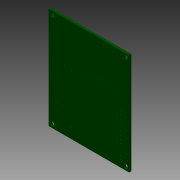
# Autodesk Inventor part: MSP-EXP430F5529LP
Saved by Autodesk Inventor 2015 SP1 (Build 190203100, 203)
## iProperties
Category: Control System
Company: Autodesk Inc.
Created: 2014-12-18
Part Number: MSP-EXP430F5529LP
Material: Generic
Document SubType Name: Modeling
Designer: Autodesk Inc.
Density: 1 g/cm^3
Appearance: Board Outline
Catalog Web Link: http://www.ti.com/tool/msp-exp430f5529lp
Vendor: Texas Instruments
Author: Autodesk Inc.
Autodesk Inventor part; units mm, degrees
ref_plane "YZ Plane" through (0, 0, 0) normal (1, 0, 0) x (0, 1, 0)
ref_plane "XZ Plane" through (0, 0, 0) normal (0, 1, 0) x (-1, 0, 0)
ref_plane "XY Plane" through (0, 0, 0) normal (0, 0, 1) x (1, 0, 0)
sketch "Sketch1" plane through (0, 0, 0) normal (0, 0, 1) x (1, 0, 0)
  line L0 (-3.81, 73.66) -> (-3.81, 0)
  line L1 (-3.81, 0) -> (54.61, 0)
  line L2 (54.61, 0) -> (54.61, 73.66)
  line L3 (54.61, 73.66) -> (-3.81, 73.66)
  circle A0 centre (2.54, 35.56) radius 0.455
  circle A1 centre (5.08, 35.56) radius 0.455
  circle A2 centre (2.54, 33.02) radius 0.455
  circle A3 centre (5.08, 33.02) radius 0.455
  circle A4 centre (2.54, 30.48) radius 0.455
  circle A5 centre (5.08, 30.48) radius 0.455
  circle A6 centre (2.54, 27.94) radius 0.455
  circle A7 centre (5.08, 27.94) radius 0.455
  circle A8 centre (2.54, 25.4) radius 0.455
  circle A9 centre (5.08, 25.4) radius 0.455
  circle A10 centre (2.54, 22.86) radius 0.455
  circle A11 centre (5.08, 22.86) radius 0.455
  circle A12 centre (2.54, 20.32) radius 0.455
  circle A13 centre (5.08, 20.32) radius 0.455
  circle A14 centre (2.54, 17.78) radius 0.455
  circle A15 centre (5.08, 17.78) radius 0.455
  circle A16 centre (2.54, 15.24) radius 0.455
  circle A17 centre (5.08, 15.24) radius 0.455
  circle A18 centre (2.54, 12.7) radius 0.455
  circle A19 centre (5.08, 12.7) radius 0.455
  circle A20 centre (2.54, 7.62) radius 0.455
  circle A21 centre (2.54, 5.08) radius 0.455
  circle A22 centre (2.54, 2.54) radius 0.455
  circle A23 centre (45.72, 35.56) radius 0.455
  circle A24 centre (48.26, 35.56) radius 0.455
  circle A25 centre (45.72, 33.02) radius 0.455
  circle A26 centre (48.26, 33.02) radius 0.455
  circle A27 centre (45.72, 30.48) radius 0.455
  circle A28 centre (48.26, 30.48) radius 0.455
  circle A29 centre (45.72, 27.94) radius 0.455
  circle A30 centre (48.26, 27.94) radius 0.455
  circle A31 centre (45.72, 25.4) radius 0.455
  circle A32 centre (48.26, 25.4) radius 0.455
  circle A33 centre (45.72, 22.86) radius 0.455
  circle A34 centre (48.26, 22.86) radius 0.455
  circle A35 centre (45.72, 20.32) radius 0.455
  circle A36 centre (48.26, 20.32) radius 0.455
  circle A37 centre (45.72, 17.78) radius 0.455
  circle A38 centre (48.26, 17.78) radius 0.455
  circle A39 centre (45.72, 15.24) radius 0.455
  circle A40 centre (48.26, 15.24) radius 0.455
  circle A41 centre (45.72, 12.7) radius 0.455
  circle A42 centre (48.26, 12.7) radius 0.455
  circle A43 centre (48.26, 7.62) radius 0.455
  circle A44 centre (48.26, 5.08) radius 0.455
  circle A45 centre (48.26, 2.54) radius 0.455
  circle A46 centre (27.94, 48.26) radius 0.455
  circle A47 centre (27.94, 45.72) radius 0.455
  circle A48 centre (30.48, 48.26) radius 0.455
  circle A49 centre (30.48, 45.72) radius 0.455
  circle A50 centre (25.4, 45.72) radius 0.455
  circle A51 centre (25.4, 48.26) radius 0.455
  circle A52 centre (45.72, 48.26) radius 0.455
  circle A53 centre (45.72, 45.72) radius 0.455
  circle A54 centre (43.18, 48.26) radius 0.455
  circle A55 centre (43.18, 45.72) radius 0.455
  circle A56 centre (48.26, 48.26) radius 0.455
  circle A57 centre (48.26, 45.72) radius 0.455
  circle A58 centre (40.64, 48.26) radius 0.455
  circle A59 centre (40.64, 45.72) radius 0.455
  circle A60 centre (38.1, 48.26) radius 0.455
  circle A61 centre (38.1, 45.72) radius 0.455
  circle A62 centre (35.56, 48.26) radius 0.455
  circle A63 centre (35.56, 45.72) radius 0.455
  circle A64 centre (33.02, 48.29) radius 0.455
  circle A65 centre (33.02, 45.75) radius 0.455
  circle A66 centre (25.4, 5.08) radius 0.455
  circle A67 centre (25.4, 2.54) radius 0.455
  circle A68 centre (12.7, 7.62) radius 0.51
  circle A69 centre (12.7, 2.62) radius 0.51
  circle A70 centre (38.1, 7.62) radius 0.51
  circle A71 centre (38.1, 2.62) radius 0.51
  circle A72 centre (2.54, 43.18) radius 0.51
  circle A73 centre (7.54, 43.18) radius 0.51
  circle A74 centre (12.7, 43.18) radius 0.51
  circle A75 centre (17.7, 43.18) radius 0.51
  circle A76 centre (48.26, 71.12) radius 0.455
  circle A77 centre (45.72, 71.12) radius 0.455
  circle A78 centre (43.18, 71.12) radius 0.455
  circle A79 centre (40.64, 71.12) radius 0.455
  circle A80 centre (38.1, 71.12) radius 0.455
  circle A81 centre (35.56, 71.12) radius 0.455
  circle A82 centre (33.02, 71.12) radius 0.455
  circle A83 centre (-1.27, 71.12) radius 1.5875
  circle A84 centre (52.07, 71.12) radius 1.5875
  circle A85 centre (52.07, 2.54) radius 1.5875
  circle A86 centre (-1.27, 2.54) radius 1.5875
  circle A87 centre (17.9832, 60.833) radius 0.1524
  circle A88 centre (20.6248, 63.246) radius 0.1524
  circle A89 centre (15.367, 60.7314) radius 0.1524
  circle A90 centre (24.0538, 66.3448) radius 0.1524
  circle A91 centre (17.526, 59.8932) radius 0.1524
  circle A92 centre (20.0406, 61.2394) radius 0.1524
  circle A93 centre (14.2748, 61.087) radius 0.1524
  circle A94 centre (21.59, 62.865) radius 0.1524
  circle A95 centre (25.019, 65.786) radius 0.1524
  circle A96 centre (35.941, 25.4762) radius 0.1524
  circle A97 centre (22.86, 39.9542) radius 0.1524
  circle A98 centre (25.7302, 42.2656) radius 0.1524
  circle A99 centre (16.5354, 15.0114) radius 0.1524
  circle A100 centre (38.4048, 17.018) radius 0.1524
  circle A101 centre (16.764, 22.5044) radius 0.1524
  circle A102 centre (5.3848, 10.4648) radius 0.1524
  circle A103 centre (10.414, 10.5156) radius 0.1524
  circle A104 centre (38.2778, 10.8712) radius 0.1524
  circle A105 centre (23.6982, 39.1668) radius 0.1524
  circle A106 centre (25.8826, 41.0718) radius 0.1524
  circle A107 centre (7.1628, 39.878) radius 0.1524
  circle A108 centre (7.1628, 37.6682) radius 0.1524
  circle A109 centre (26.4414, 63.4238) radius 0.1524
  circle A110 centre (28.9052, 62.103) radius 0.1524
  circle A111 centre (32.7152, 54.8386) radius 0.1524
  circle A112 centre (30.8356, 57.404) radius 0.1524
  circle A113 centre (25.7302, 62.5348) radius 0.1524
  circle A114 centre (28.5242, 61.214) radius 0.1524
  circle A115 centre (31.7754, 54.0258) radius 0.1524
  circle A116 centre (29.972, 56.4896) radius 0.1524
  circle A117 centre (17.5768, 50.4444) radius 0.1524
  circle A118 centre (19.6088, 52.451) radius 0.1524
  circle A119 centre (38.4556, 63.754) radius 0.1524
  circle A120 centre (40.4114, 59.9186) radius 0.1524
  circle A121 centre (41.6814, 58.6232) radius 0.1524
  circle A122 centre (38.7096, 61.6204) radius 0.1524
  circle A123 centre (38.7858, 52.4764) radius 0.1524
  circle A124 centre (36.068, 51.6128) radius 0.1524
  circle A125 centre (32.258, 52.4764) radius 0.1524
  circle A126 centre (27.432, 52.451) radius 0.1524
  circle A127 centre (29.591, 52.4764) radius 0.1524
  circle A128 centre (31.0134, 51.2572) radius 0.1524
  circle A129 centre (16.7386, 51.308) radius 0.1524
  circle A130 centre (18.9992, 53.5178) radius 0.1524
  circle A131 centre (43.7134, 52.1208) radius 0.1524
  circle A132 centre (28.3718, 70.5612) radius 0.1524
  circle A133 centre (42.5704, 50.1142) radius 0.1524
  circle A134 centre (36.2966, 50.5714) radius 0.1524
  circle A135 centre (28.4734, 68.6308) radius 0.1524
  circle A136 centre (30.2768, 66.7512) radius 0.1524
  circle A137 centre (30.5562, 62.103) radius 0.1524
  circle A138 centre (7.0866, 55.4736) radius 0.1524
  circle A139 centre (11.557, 64.5922) radius 0.1524
  circle A140 centre (20.066, 67.5132) radius 0.1524
  circle A141 centre (13.97, 67.4116) radius 0.1524
  circle A142 centre (12.573, 67.4116) radius 0.1524
  circle A143 centre (13.1826, 62.484) radius 0.1524
  circle A144 centre (13.1826, 60.5536) radius 0.1524
  circle A145 centre (7.2898, 66.0146) radius 0.1524
  circle A146 centre (6.7818, 64.516) radius 0.1524
  circle A147 centre (7.3914, 68.2244) radius 0.1524
  circle A148 centre (3.6576, 66.9798) radius 0.1524
  circle A149 centre (6.0452, 58.42) radius 0.1524
  circle A150 centre (4.064, 54.2544) radius 0.1524
  circle A151 centre (28.3718, 59.9694) radius 0.1524
  circle A152 centre (11.557, 63.4746) radius 0.1524
  circle A153 centre (23.1902, 69.6468) radius 0.1524
  circle A154 centre (27.3812, 69.6468) radius 0.1524
  circle A155 centre (28.3464, 71.7042) radius 0.1524
  circle A156 centre (42.6212, 5.715) radius 0.1524
  circle A157 centre (7.6962, 5.1308) radius 0.1524
  circle A158 centre (22.1234, 1.9304) radius 0.1524
  circle A159 centre (32.1564, 1.905) radius 0.1524
  circle A160 centre (16.9418, 19.2786) radius 0.1524
  circle A161 centre (11.0744, 24.5618) radius 0.1524
  circle A162 centre (32.893, 58.8772) radius 0.1524
  circle A163 centre (34.4678, 62.6872) radius 0.1524
  circle A164 centre (31.9786, 61.9506) radius 0.1524
  circle A165 centre (42.799, 51.2318) radius 0.1524
  circle A166 centre (45.8216, 61.6712) radius 0.1524
  circle A167 centre (44.958, 62.5094) radius 0.1524
  circle A168 centre (11.5062, 67.7164) radius 0.1524
  circle A169 centre (14.7066, 57.7088) radius 0.1524
  circle A170 centre (18.288, 57.7342) radius 0.1524
  circle A171 centre (18.288, 56.3118) radius 0.1524
  circle A172 centre (14.7066, 56.3118) radius 0.1524
  circle A173 centre (30.8102, 32.2326) radius 0.1524
  circle A174 centre (28.1432, 37.7444) radius 0.1524
  circle A175 centre (26.797, 37.7444) radius 0.1524
  circle A176 centre (26.6192, 30.6324) radius 0.1524
  circle A177 centre (23.5712, 38.2016) radius 0.1524
  circle A178 centre (34.3154, 32.639) radius 0.1524
  circle A179 centre (35.8902, 24.1554) radius 0.1524
  circle A180 centre (19.685, 44.6532) radius 0.1524
  circle A181 centre (23.4188, 44.6786) radius 0.1524
  circle A182 centre (20.3962, 42.5196) radius 0.1524
  circle A183 centre (10.4902, 45.7454) radius 0.1524
  circle A184 centre (21.0058, 13.3096) radius 0.1524
  circle A185 centre (18.5928, 15.3924) radius 0.1524
  circle A186 centre (14.4272, 18.6944) radius 0.1524
  circle A187 centre (10.9728, 18.6944) radius 0.1524
  circle A188 centre (45.8978, 63.3222) radius 0.1524
  circle A189 centre (48.9966, 58.9534) radius 0.1524
  circle A190 centre (45.1612, 57.3024) radius 0.1524
  circle A191 centre (45.6692, 55.6768) radius 0.1524
  circle A192 centre (34.544, 66.2432) radius 0.1524
  circle A193 centre (30.3784, 54.1274) radius 0.1524
  circle A194 centre (38.6842, 60.0456) radius 0.1524
  circle A195 centre (35.7378, 57.0992) radius 0.1524
  circle A196 centre (37.5666, 55.2704) radius 0.1524
  circle A197 centre (41.5798, 57.0484) radius 0.1524
  circle A198 centre (40.6146, 57.9628) radius 0.1524
  circle A199 centre (39.6748, 58.9026) radius 0.1524
  circle A200 centre (37.7444, 59.0804) radius 0.1524
  circle A201 centre (36.7792, 58.0898) radius 0.1524
  circle A202 centre (38.608, 58.0898) radius 0.1524
  circle A203 centre (37.6428, 57.0738) radius 0.1524
  circle A204 centre (36.6522, 56.2356) radius 0.1524
  circle A205 centre (38.6334, 54.1274) radius 0.1524
  circle A206 centre (39.5732, 55.0926) radius 0.1524
  circle A207 centre (40.6146, 56.134) radius 0.1524
  circle A208 centre (39.6748, 57.0738) radius 0.1524
  circle A209 centre (38.6334, 56.0832) radius 0.1524
  circle A210 centre (45.6184, 66.8782) radius 0.1524
  circle A211 centre (43.3578, 63.7032) radius 0.1524
  circle A212 centre (42.037, 63.6016) radius 0.1524
  circle A213 centre (31.8008, 65.5828) radius 0.1524
  circle A214 centre (24.2316, 68.3514) radius 0.1524
  circle A215 centre (24.2316, 67.2592) radius 0.1524
  circle A216 centre (24.2824, 63.8556) radius 0.1524
  circle A217 centre (24.2824, 64.9732) radius 0.1524
  circle A218 centre (22.1742, 61.341) radius 0.1524
  circle A219 centre (23.5458, 61.341) radius 0.1524
  circle A220 centre (23.4696, 57.7596) radius 0.1524
  circle A221 centre (22.1234, 57.7596) radius 0.1524
  circle A222 centre (12.5476, 69.9516) radius 0.1524
  circle A223 centre (17.7292, 68.0466) radius 0.1524
  circle A224 centre (16.4338, 68.6054) radius 0.1524
  circle A225 centre (2.3114, 55.245) radius 0.1524
  circle A226 centre (-1.4478, 38.1254) radius 0.1524
  circle A227 centre (-2.3622, 43.1546) radius 0.1524
  circle A228 centre (-0.4826, 48.5902) radius 0.1524
  circle A229 centre (5.0292, 45.7454) radius 0.1524
  circle A230 centre (15.1892, 45.6184) radius 0.1524
  circle A231 centre (15.8242, 40.5384) radius 0.1524
  circle A232 centre (43.1292, 10.9474) radius 0.1524
  circle A233 centre (10.6426, 35.4584) radius 0.1524
  circle A234 centre (14.4272, 36.0934) radius 0.1524
  circle A235 centre (17.526, 36.2204) radius 0.1524
  circle A236 centre (24.5872, 33.6804) radius 0.1524
  circle A237 centre (20.2184, 29.6418) radius 0.1524
  circle A238 centre (23.9522, 29.6164) radius 0.1524
  circle A239 centre (22.1488, 26.5938) radius 0.1524
  circle A240 centre (37.2872, 23.7744) radius 0.1524
  circle A241 centre (29.4132, 26.9494) radius 0.1524
  circle A242 centre (31.0642, 34.6964) radius 0.1524
  circle A243 centre (28.0162, 41.1734) radius 0.1524
  circle A244 centre (31.6992, 43.9674) radius 0.1524
  circle A245 centre (41.9354, 34.1122) radius 0.1524
  circle A246 centre (48.0568, 38.0746) radius 0.1524
  circle A247 centre (33.4772, 31.7754) radius 0.1524
  circle A248 centre (34.3408, 41.529) radius 0.1524
  circle A249 centre (34.3408, 37.2872) radius 0.1524
  circle A250 centre (41.0972, 37.3634) radius 0.1524
  circle A251 centre (39.7002, 42.4434) radius 0.1524
  circle A252 centre (47.0662, 43.5864) radius 0.1524
  circle A253 centre (44.5262, 39.0144) radius 0.1524
  circle A254 centre (43.2054, 31.8008) radius 0.1524
  circle A255 centre (50.8762, 37.1094) radius 0.1524
  circle A256 centre (50.546, 49.6316) radius 0.1524
  circle A257 centre (46.8884, 53.6702) radius 0.1524
  circle A258 centre (50.6222, 53.6194) radius 0.1524
  circle A259 centre (49.9872, 56.6674) radius 0.1524
  circle A260 centre (50.4952, 60.7314) radius 0.1524
  circle A261 centre (50.6222, 65.4304) radius 0.1524
  circle A262 centre (49.8602, 67.7164) radius 0.1524
  circle A263 centre (50.4952, 63.0174) radius 0.1524
  circle A264 centre (46.5582, 66.1924) radius 0.1524
  circle A265 centre (39.3192, 66.0654) radius 0.1524
  circle A266 centre (39.1922, 67.7164) radius 0.1524
  circle A267 centre (37.7952, 67.8434) radius 0.1524
  circle A268 centre (32.8422, 67.4624) radius 0.1524
  circle A269 centre (31.5722, 66.8274) radius 0.1524
  circle A270 centre (35.7632, 62.2554) radius 0.1524
  circle A271 centre (38.5318, 66.8274) radius 0.1524
  circle A272 centre (36.7792, 70.1294) radius 0.1524
  circle A273 centre (41.8592, 70.1294) radius 0.1524
  circle A274 centre (21.6662, 72.1614) radius 0.1524
  circle A275 centre (21.2852, 70.0024) radius 0.1524
  circle A276 centre (24.4602, 62.5094) radius 0.1524
  circle A277 centre (26.6192, 56.6674) radius 0.1524
  circle A278 centre (27.5082, 67.7164) radius 0.1524
  circle A279 centre (26.8732, 58.4454) radius 0.1524
  circle A280 centre (22.8092, 54.6354) radius 0.1524
  circle A281 centre (23.4442, 55.6514) radius 0.1524
  circle A282 centre (19.6342, 57.8104) radius 0.1524
  circle A283 centre (19.8882, 54.7624) radius 0.1524
  circle A284 centre (23.4696, 51.6128) radius 0.1524
  circle A285 centre (20.9042, 51.4604) radius 0.1524
  circle A286 centre (46.9392, 50.3936) radius 0.1524
  circle A287 centre (17.3482, 48.9204) radius 0.1524
  circle A288 centre (18.8722, 48.0314) radius 0.1524
  circle A289 centre (26.7462, 54.6354) radius 0.1524
  circle A290 centre (19.7612, 45.9994) radius 0.1524
  circle A291 centre (18.5928, 46.355) radius 0.1524
  circle A292 centre (15.5702, 49.3014) radius 0.1524
  circle A293 centre (14.0462, 49.5554) radius 0.1524
  circle A294 centre (14.3002, 52.2224) radius 0.1524
  circle A295 centre (16.2052, 52.4764) radius 0.1524
  circle A296 centre (13.6652, 53.4924) radius 0.1524
  circle A297 centre (13.0302, 56.5404) radius 0.1524
  circle A298 centre (10.6172, 59.5884) radius 0.1524
  circle A299 centre (9.7282, 58.5724) radius 0.1524
  circle A300 centre (8.4582, 58.1914) radius 0.1524
  circle A301 centre (9.2202, 59.8424) radius 0.1524
  circle A302 centre (9.2202, 61.4934) radius 0.1524
  circle A303 centre (8.7122, 62.8904) radius 0.1524
  circle A304 centre (6.9342, 62.5094) radius 0.1524
  circle A305 centre (5.5372, 62.5094) radius 0.1524
  circle A306 centre (4.3942, 62.2554) radius 0.1524
  circle A307 centre (3.5052, 61.3664) radius 0.1524
  circle A308 centre (3.5052, 60.0964) radius 0.1524
  circle A309 centre (19.6342, 72.6694) radius 0.1524
  circle A310 centre (13.0302, 68.8594) radius 0.1524
  circle A311 centre (13.7922, 72.7964) radius 0.1524
  circle A312 centre (1.3462, 61.4934) radius 0.1524
  circle A313 centre (1.3462, 59.9694) radius 0.1524
  circle A314 centre (1.905, 69.9516) radius 0.1524
  circle A315 centre (-2.2606, 53.975) radius 0.1524
  circle A316 centre (-2.4638, 56.9214) radius 0.1524
  circle A317 centre (0.635, 67.8434) radius 0.1524
  circle A318 centre (-0.2794, 66.4972) radius 0.1524
  circle A319 centre (-2.0066, 50.1396) radius 0.1524
  circle A320 centre (-1.2192, 60.6806) radius 0.1524
  circle A321 centre (-0.1778, 64.9986) radius 0.1524
  circle A322 centre (-0.5588, 55.9054) radius 0.1524
  circle A323 centre (-0.4826, 53.8988) radius 0.1524
  circle A324 centre (-0.5334, 52.2224) radius 0.1524
  circle A325 centre (-0.254, 50.6476) radius 0.1524
  circle A326 centre (0.8382, 49.4284) radius 0.1524
  circle A327 centre (6.5532, 49.4284) radius 0.1524
  circle A328 centre (11.2522, 49.3014) radius 0.1524
  circle A329 centre (-1.0668, 34.0614) radius 0.1524
  circle A330 centre (-0.3048, 46.0502) radius 0.1524
  circle A331 centre (-1.0668, 31.6484) radius 0.1524
  circle A332 centre (-1.0668, 28.9814) radius 0.1524
  circle A333 centre (-1.1938, 26.5684) radius 0.1524
  circle A334 centre (-1.0668, 23.9014) radius 0.1524
  circle A335 centre (-1.1938, 21.717) radius 0.1524
  circle A336 centre (-1.1176, 19.1008) radius 0.1524
  circle A337 centre (-1.016, 16.4084) radius 0.1524
  circle A338 centre (-1.3208, 13.7668) radius 0.1524
  circle A339 centre (-0.3048, 10.5664) radius 0.1524
  circle A340 centre (0.7112, 9.2964) radius 0.1524
  circle A341 centre (6.223, 9.017) radius 0.1524
  circle A342 centre (18.6944, 9.9822) radius 0.1524
  circle A343 centre (46.5582, 6.3754) radius 0.1524
  circle A344 centre (49.7332, 10.3124) radius 0.1524
  circle A345 centre (51.8922, 11.2014) radius 0.1524
  circle A346 centre (51.5112, 13.8684) radius 0.1524
  circle A347 centre (51.1302, 16.4084) radius 0.1524
  circle A348 centre (51.1302, 18.6944) radius 0.1524
  circle A349 centre (51.0032, 21.4884) radius 0.1524
  circle A350 centre (51.0032, 24.0284) radius 0.1524
  circle A351 centre (51.1302, 26.8224) radius 0.1524
  circle A352 centre (51.0032, 28.9814) radius 0.1524
  circle A353 centre (51.0032, 31.6484) radius 0.1524
  circle A354 centre (51.0032, 34.0614) radius 0.1524
  circle A355 centre (43.0022, 16.5354) radius 0.1524
  circle A356 centre (33.4772, 27.0764) radius 0.1524
  circle A357 centre (37.0332, 26.3144) radius 0.1524
  circle A358 centre (34.4932, 18.5674) radius 0.1524
  circle A359 centre (27.7622, 27.7114) radius 0.1524
  circle A360 centre (27.2796, 20.5994) radius 0.1524
  circle A361 centre (48.8442, 40.3352) radius 0.1524
  circle A362 centre (20.2438, 11.9126) radius 0.1524
  circle A363 centre (28.8544, 20.0914) radius 0.1524
  circle A364 centre (21.4884, 21.5392) radius 0.1524
  circle A365 centre (22.1488, 23.3426) radius 0.1524
  circle A366 centre (31.9278, 18.542) radius 0.1524
  circle A367 centre (42.8752, 23.9014) radius 0.1524
  circle A368 centre (17.2212, 17.6784) radius 0.1524
  circle A369 centre (19.5072, 14.7574) radius 0.1524
  circle A370 centre (14.1986, 13.8176) radius 0.1524
  circle A371 centre (17.2212, 4.4704) radius 0.1524
  circle A372 centre (9.779, 1.2954) radius 0.1524
  circle A373 centre (27.6352, 2.5654) radius 0.1524
  circle A374 centre (34.1122, 3.5814) radius 0.1524
  circle A375 centre (27.813, 6.0198) radius 0.1524
  circle A376 centre (40.0812, 5.1054) radius 0.1524
  circle A377 centre (9.0932, 36.7284) radius 0.1524
  circle A378 centre (53.2892, 6.5024) radius 0.1524
  circle A379 centre (-2.7178, 6.8834) radius 0.1524
  circle A380 centre (12.8016, 15.2146) radius 0.1524
  circle A381 centre (11.0998, 15.5448) radius 0.1524
  circle A382 centre (14.605, 15.7226) radius 0.1524
  circle A383 centre (14.6812, 17.2974) radius 0.1524
  circle A384 centre (12.7254, 20.32) radius 0.1524
  circle A385 centre (11.176, 17.3228) radius 0.1524
  circle A386 centre (15.1892, 22.6314) radius 0.1524
  circle A387 centre (23.4442, 33.6804) radius 0.1524
  circle A388 centre (1.4224, 31.7246) radius 0.1524
  circle A389 centre (30.3022, 39.3954) radius 0.1524
  circle A390 centre (33.2232, 34.0614) radius 0.1524
  circle A391 centre (15.367, 10.0076) radius 0.1524
  circle A392 centre (15.7734, 64.7192) radius 0.1524
  circle A393 centre (18.2626, 64.7192) radius 0.1524
  circle A394 centre (17.018, 64.7192) radius 0.1524
  circle A395 centre (15.7734, 65.9638) radius 0.1524
  circle A396 centre (18.2626, 65.9638) radius 0.1524
  circle A397 centre (17.018, 65.9638) radius 0.1524
  circle A398 centre (15.7734, 63.4492) radius 0.1524
  circle A399 centre (18.2626, 63.4492) radius 0.1524
  circle A400 centre (17.018, 63.4492) radius 0.1524
  circle A401 centre (40.0812, 9.652) radius 0.1524
  circle A402 centre (31.9278, 50.2158) radius 0.1524
  circle A403 centre (34.6964, 53.0606) radius 0.1524
  circle A404 centre (49.0982, 50.5206) radius 0.1524
  circle A405 centre (26.3906, 51.4858) radius 0.1524
  circle A406 centre (52.6796, 37.8714) radius 0.1524
  circle A407 centre (1.3716, 34.3408) radius 0.1524
  circle A408 centre (1.3208, 29.1592) radius 0.1524
  circle A409 centre (1.3208, 26.6954) radius 0.1524
  circle A410 centre (11.0236, 11.938) radius 0.1524
  circle A411 centre (7.874, 13.9192) radius 0.1524
  circle A412 centre (1.2192, 13.9954) radius 0.1524
  circle A413 centre (15.9512, 23.9522) radius 0.1524
  circle A414 centre (11.6586, 13.7922) radius 0.1524
  circle A415 centre (15.24, 11.7856) radius 0.1524
  circle A416 centre (2.1844, 51.9938) radius 0.1524
  circle A417 centre (4.826, 51.9938) radius 0.1524
  circle A418 centre (10.16, 52.8066) radius 0.1524
  circle A419 centre (4.2672, 6.2484) radius 0.1524
  circle A420 centre (10.6172, 5.2324) radius 0.1524
  circle A421 centre (4.3942, 9.4234) radius 0.1524
  circle A422 centre (45.2882, 68.0212) radius 0.1524
  circle A423 centre (34.29, 68.453) radius 0.1524
  circle A424 centre (45.466, 69.1388) radius 0.1524
  circle A425 centre (33.6296, 69.1388) radius 0.1524
  circle A426 centre (2.8956, 69.2404) radius 0.1524
  circle A427 centre (13.6906, 64.7192) radius 0.1524
  circle A428 centre (14.097, 62.103) radius 0.1524
  circle A429 centre (4.2672, 70.485) radius 0.1524
  circle A430 centre (9.0932, 70.485) radius 0.1524
  circle A431 centre (10.4648, 69.2404) radius 0.1524
  circle A432 centre (11.2014, 72.7964) radius 0.1524
  circle A433 centre (10.3632, 71.628) radius 0.1524
  circle A434 centre (2.9972, 71.628) radius 0.1524
  circle A435 centre (2.159, 72.7964) radius 0.1524
  circle A436 centre (5.842, 72.1868) radius 0.1524
  circle A437 centre (7.5692, 72.1868) radius 0.1524
  circle A438 centre (23.4442, 12.7762) radius 0.1524
  circle A439 centre (20.5486, 9.9314) radius 0.1524
  circle A440 centre (20.5486, 7.2136) radius 0.1524
  circle A441 centre (22.1742, 10.0076) radius 0.1524
  circle A442 centre (25.908, 12.446) radius 0.1524
  circle A443 centre (26.162, 10.033) radius 0.1524
  circle A444 centre (8.636, 16.51) radius 0.1524
  circle A445 centre (6.223, 16.51) radius 0.1524
  circle A446 centre (23.368, 10.033) radius 0.1524
  circle A447 centre (23.876, 16.891) radius 0.1524
  circle A448 centre (37.592, 35.052) radius 0.1524
  circle A449 centre (34.29, 34.417) radius 0.1524
  circle A450 centre (23.495, 24.13) radius 0.1524
  circle A451 centre (29.591, 24.638) radius 0.1524
  circle A452 centre (25.5524, 8.5344) radius 0.1524
  circle A453 centre (25.4, 19.939) radius 0.1524
  circle A454 centre (44.069, 29.464) radius 0.1524
  circle A455 centre (40.767, 29.464) radius 0.1524
  circle A456 centre (27.686, 11.557) radius 0.1524
  circle A457 centre (26.416, 16.129) radius 0.1524
  circle A458 centre (28.194, 16.891) radius 0.1524
  circle A459 centre (29.718, 11.684) radius 0.1524
  circle A460 centre (21.9202, 25.1968) radius 0.1524
  circle A461 centre (16.2306, 26.5938) radius 0.1524
  circle A462 centre (8.89, 19.558) radius 0.1524
  circle A463 centre (3.81, 19.05) radius 0.1524
  circle A464 centre (38.1, 22.606) radius 0.1524
  circle A465 centre (44.069, 23.622) radius 0.1524
  circle A466 centre (37.719, 21.59) radius 0.1524
  circle A467 centre (43.8404, 21.844) radius 0.1524
  circle A468 centre (15.5448, 25.8826) radius 0.1524
  circle A469 centre (20.3454, 25.2222) radius 0.1524
  circle A470 centre (8.9916, 21.3106) radius 0.1524
  circle A471 centre (3.937, 21.59) radius 0.1524
  circle A472 centre (21.7678, 29.2608) radius 0.1524
  circle A473 centre (23.4442, 26.5684) radius 0.1524
  circle A474 centre (11.3792, 33.909) radius 0.1524
  circle A475 centre (13.4366, 31.9786) radius 0.1524
  circle A476 centre (22.5806, 29.7688) radius 0.1524
  circle A477 centre (24.384, 26.9748) radius 0.1524
  circle A478 centre (12.0142, 34.7218) radius 0.1524
  circle A479 centre (14.605, 32.131) radius 0.1524
  circle A480 centre (21.082, 27.051) radius 0.1524
  circle A481 centre (16.637, 27.432) radius 0.1524
  circle A482 centre (16.002, 28.321) radius 0.1524
  circle A483 centre (20.32, 27.813) radius 0.1524
  circle A484 centre (36.068, 19.558) radius 0.1524
  circle A485 centre (44.323, 18.923) radius 0.1524
  circle A486 centre (37.338, 20.193) radius 0.1524
  circle A487 centre (44.069, 20.447) radius 0.1524
  circle A488 centre (30.861, 23.1902) radius 0.1524
  circle A489 centre (24.638, 9.1694) radius 0.1524
  circle A490 centre (24.13, 20.701) radius 0.1524
  circle A491 centre (24.257, 22.733) radius 0.1524
  circle A492 centre (23.368, 23.114) radius 0.1524
  circle A493 centre (30.381, 24.031) radius 0.1524
  circle A494 centre (23.368, 20.066) radius 0.1524
  circle A495 centre (24.511, 10.16) radius 0.1524
  circle A496 centre (42.9768, 21.082) radius 0.1524
  circle A497 centre (36.449, 20.828) radius 0.1524
  circle A498 centre (37.973, 29.21) radius 0.1524
  circle A499 centre (38.6334, 31.9024) radius 0.1524
  circle A500 centre (37.973, 32.639) radius 0.1524
  circle A501 centre (36.957, 29.4386) radius 0.1524
  circle A502 centre (30.48, 25.019) radius 0.1524
  circle A503 centre (25.781, 20.828) radius 0.1524
  circle A504 centre (26.543, 9.017) radius 0.1524
  circle A505 centre (24.511, 24.384) radius 0.1524
  circle A506 centre (13.462, 30.353) radius 0.1524
  circle A507 centre (8.89, 34.29) radius 0.1524
  circle A508 centre (6.096, 34.163) radius 0.1524
  circle A509 centre (11.811, 29.785) radius 0.1524
  circle A510 centre (7.239, 29.21) radius 0.1524
  circle A511 centre (29.4386, 29.2608) radius 0.1524
  circle A512 centre (34.163, 29.337) radius 0.1524
  circle A513 centre (35.9918, 29.21) radius 0.1524
  circle A514 centre (37.2618, 31.877) radius 0.1524
  circle A515 centre (38.227, 26.924) radius 0.1524
  circle A516 centre (42.164, 26.797) radius 0.1524
  circle A517 centre (34.342, 27.761) radius 0.1524
  circle A518 centre (36.576, 27.305) radius 0.1524
  circle A519 centre (28.194, 29.2862) radius 0.1524
  circle A520 centre (33.7312, 30.226) radius 0.1524
  circle A521 centre (11.7602, 39.9034) radius 0.1524
  circle A522 centre (11.7602, 36.8808) radius 0.1524
  circle A523 centre (42.418, 25.908) radius 0.1524
  circle A524 centre (38.6842, 26.1112) radius 0.1524
  circle A525 centre (24.4602, 43.1292) radius 0.1524
  circle A526 centre (21.8694, 41.1988) radius 0.1524
  circle A527 centre (27.7368, 30.2514) radius 0.1524
  circle A528 centre (32.5882, 30.9118) radius 0.1524
  circle A529 centre (42.037, 42.799) radius 0.1524
  circle A530 centre (44.2468, 42.799) radius 0.1524
  constraints: 531 centre point, 8 end point
extrude "CS_LaunchpadModule_MSP-EXP430F5529LP" add sketch "Sketch1" along normal blind 1.6
body "Solid1"
